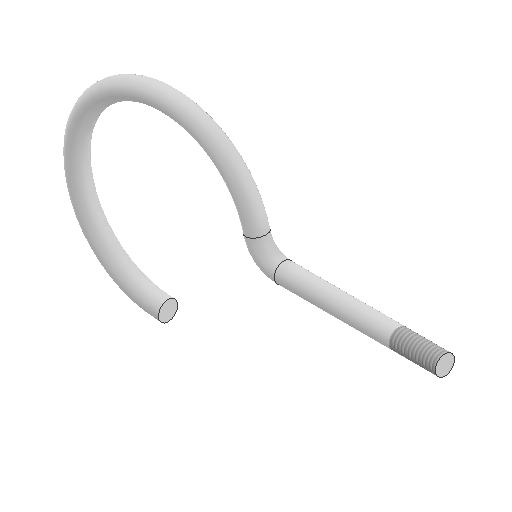
# Autodesk Inventor part: Gancho
Saved by Autodesk Inventor 2026.1 (Build 301233000, 233)
## iProperties
Created: 2025-08-11
Part Number: Gancho
Material: Genérico
Document SubType Name: Modeling
Designer: gianm
Density: 1 g/cm^3
Appearance: Valor por defecto
Author: gianm
Autodesk Inventor part; units mm, degrees
ref_plane "YZ Plane" through (0, 0, 0) normal (1, 0, 0) x (0, 1, 0)
ref_plane "XZ Plane" through (0, 0, 0) normal (0, 1, 0) x (-1, 0, 0)
ref_plane "XY Plane" through (0, 0, 0) normal (0, 0, 1) x (1, 0, 0)
sketch "Boceto1" plane through (0, 0, 0) normal (0, 0, 1) x (1, 0, 0)
  arc A0 (12.6427, 3.0271) -> (0, -13) centre (0, 0) ccw
  arc A1 (12.6427, 3.0271) -> (14.8955, 1.25) centre (14.8955, 3.5665) ccw
  line L0 (14.8955, 1.25) -> (35.6427, 1.25)
  line L1 (35.6427, 1.25) -> (35.6427, -1.25) construction
  line L2 (35.6427, 0) -> (-13, 0) construction
  dimension "d0" = 2.5
  dimension "d1" = 13
  dimension "d2" = 23
  constraints: 6 end point, 5 point on circle, 2 centre point, 2 horizontal, 2 tangent, 1 coincident, 1 midpoint, 1 point on line, 1 vertical, 1 vertical alignment
  measures "d0" distance of L0.end L1.end
  measures "d1" radius of A0
  measures "d2" horizontal distance of L0.end A0.start
ref_plane "Plano de trabajo1" through (35.6427, 1.25, 0) normal (1, 0, 0) x (0, 1, 0)
sketch "Boceto3" plane through (35.6427, 1.25, 0) normal (1, 0, 0) x (0, 1, 0)
  circle A0 centre (-1.25, 0) radius 1.25
  constraints: 1 centre point, 1 coincident
sweep "Barrido1" add profiles "Boceto3" path "Boceto1" path curves L0 A1 A0
thread "Rosca1"
